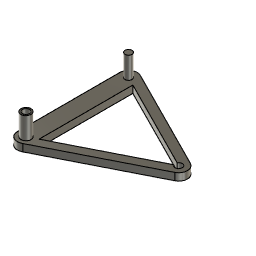
escapement_linkage v6 (Autodesk Fusion 360 archive; units mm, degrees)
design "frame"
Autodesk Fusion 360 part; units mm, degrees
sketch "Sketch1" plane through (0, 0, 0) normal (0, 0, 1) x (1, 0, 0)
  circle A0 centre (0, 0) radius 50
  circle A1 centre (0, 0) radius 37.5
  circle A2 centre (0, 0) radius 33
  circle A3 centre (0, 0) radius 10
  circle A4 centre (0, 0) radius 3.5
  line L0 (0, 0) -> (-100.3747, 100.3747)
  line L1 (0, 0) -> (141.9513, 0) construction
  line L2 (0, 0) -> (0, 143.4713)
  line L3 (-35.3553, 35.3553) -> (13.4462, 84.1569)
  circle A5 centre (0, 70.7107) radius 6
  circle A6 centre (0, 70.7107) radius 2.5
  circle A7 centre (0, 120.7107) radius 6
  line L4 (5.9996, 70.7836) -> (5.9996, 120.7836)
  line L5 (-5.9996, 70.7836) -> (-5.9996, 120.7836)
  line L6 (0, 0) -> (-100.7319, 104.311)
  line L7 (5.9996, 120.7836) -> (5.9996, 95.7836)
  line L8 (-3.0629, 75.87) -> (-47.5954, 50.1551)
  line L9 (-46.505, 50.7838) -> (-53.2901, 46.8719)
  line L10 (46.505, 50.7838) -> (53.2901, 46.8719)
  line L11 (3.0629, 75.87) -> (49.2585, 49.2366)
  line L12 (-53.2901, 46.8719) -> (-50.2933, 41.6739)
  line L13 (-50.2933, 41.6739) -> (0, 64.7107)
  line L14 (50.2933, 41.6739) -> (0, 64.7107)
  line L15 (53.2901, 46.8719) -> (50.2933, 41.6739)
  line L16 (-35.3553, 35.3553) -> (55, 35.3553)
  line L17 (-35.3553, 35.3553) -> (-52, 35.3553)
  line L18 (35.3553, 35.3553) -> (35.3553, 40.6)
  line L19 (35.3553, 35.3553) -> (35.3553, 30.1107)
  line L20 (0, 0) -> (-100.7319, 104.311)
  line L21 (0, 0) -> (-105.6852, 95.1594)
  line L22 (0, 0) -> (142.2568, 0) construction
  circle A8 centre (0, 70.7107) radius 52.618
  circle A9 centre (0, 70.7107) radius 49.5405
  circle A10 centre (34.4479, 35.6863) radius 0.4
  line L23 (25.0068, 27.9448) -> (34.6694, 35.3533)
  line L24 (25.0068, 27.9448) -> (0, 0)
  line L25 (0, 0) -> (19.4334, 32.4512)
  spline S0 degree 5 poles (19.4334, 32.4512) (19.6407, 32.3946) (20.0636, 32.2932) (20.7228, 32.1772) (21.6523, 32.0954) (22.9036, 32.1224) (24.2503, 32.2872) (25.6967, 32.596) (27.2397, 33.0445) (28.8713, 33.6208) (30.5824, 34.3122) (32.0089, 34.9483) (33.1088, 35.469) (33.8553, 35.8351) (34.2318, 36.0229) knots 0 0 0 0 0 0 0.1 0.2 0.3 0.4 0.5 0.6 0.7 0.8 0.9 1 1 1 1 1 1
  circle A11 centre (0, 0) radius 2.5
  point P0 (24.6678, 32.3946)
  dimension "d2" = 75
  dimension "d3" = 66
  dimension "d4" = 20
  dimension "d5" = 7
  dimension "d6" = 135
  dimension "d7" = 12
  dimension "d8" = 5
  dimension "d9" = 12
  dimension "d10" = 50
  dimension "d11" = 1
  dimension "d15" = 6
  dimension "d25" = 138
  dimension "d26" = 1
  dimension "d27" = 0.8
  dimension "d28" = 10.909
  dimension "d62" = 5
  constraint coincident A0.centre A1.centre
  constraint concentric A0 A1
  constraint concentric A1 A2
  constraint concentric A2 A3
  constraint concentric A3 A4
  constraint horizontal L1
  constraint vertical L2
  constraint coincident A0 L3.start
  constraint coincident L0 L3.start
  constraint tangent A0 L3
  constraint coincident L3 A5.centre
  constraint coincident L2 A5.centre
  constraint concentric A5 A6
  constraint coincident A5 L4.start
  constraint symmetric L2 L4.start L5.start
  constraint symmetric L2 L4.end L5.end
  constraint parallel L4 L7
  constraint perpendicular L9 L12
  constraint coincident A5 L13.end
  constraint coincident L2 L13.end
  constraint symmetric L2 L9.end L10.end
  constraint symmetric L2 L12.end L14.start
  constraint symmetric L2 L13.end L14.end
  constraint horizontal L16
  constraint horizontal L17
  constraint coincident A0 L18.start
  constraint coincident L16 L18.start
  constraint perpendicular L16 L18
  constraint symmetric L16 L18.start L19.start
  constraint symmetric L16 L18.end L19.end
  constraint horizontal L22
  constraint concentric A6 A8
  constraint concentric A5 A9
  constraint coincident A1 L23.start
  constraint coincident A9 L23.start
  constraint coincident A10 L23.end
  constraint coincident A10 S0.end
  constraint concentric A3 A11
  measures "d2" diameter of A1
  measures "d3" diameter of A2
  measures "d4" diameter of A3
  measures "d5" diameter of A4
  measures "d6" angle of L0 L1
  measures "d7" diameter of A5
  measures "d8" diameter of A6
  measures "d9" diameter of A7
  measures "d10" distance of L4.start L4.end
  measures "d11" angle of L0 L6
  measures "d15" distance of L9.end L12.end
  measures "d25" angle of L21 L22
  measures "d27" diameter of A10
  measures "d28" angle of L24 L25
  measures "d62" diameter of A11
pattern_circular "C-Pattern1" [no effect]
sketch "Sketch3" plane through (0, 0, 0) normal (0, 0, 1) x (1, 0, 0)
  circle A0 centre (80, 70.7107) radius 6
  circle A1 centre (80, 70.7107) radius 2.45
  circle A2 centre (80, -0.0003) radius 6
  line L0 (80, 70.7107) -> (80, -0.0003)
  line L1 (74, 70.7107) -> (74, -0.0003)
  line L2 (86, 67.6807) -> (86, 3.0309)
  circle A3 centre (80, 0) radius 3.5
  circle A4 centre (80, 0) radius 2.5
  circle A5 centre (54, 100) radius 3
  line L3 (80, 70.7107) -> (80, 35.3607)
  line L4 (150, 35.3607) -> (150, 47)
  line L5 (152.7047, 40.7165) -> (82.7047, 76.0665)
  line L6 (152.7047, 30.0049) -> (82.7047, -5.3451)
  circle A6 centre (150, 35.3607) radius 2.5
  line L7 (150, 47) -> (150, 32.8607)
  line L8 (150, 28.639) -> (150, 24)
  arc A7 (152.7047, 30.0049) -> (152.7047, 40.7165) centre (150, 35.3607) ccw
  line L9 (80, 35.3607) -> (86, 35.3607)
  line L10 (147.5, 35.3607) -> (150, 35.3607)
  line L11 (150, 35.3607) -> (86, 67.6807)
  line L12 (85.3558, 68.006) -> (80, 70.7107)
  line L13 (80, 0) -> (85.3554, 2.7053)
  line L14 (86, 3.0309) -> (150, 35.3607)
  point P0 (0, 70.7107)
  dimension "d68" = 12
  dimension "d71" = 4.9
  dimension "d73" = 12
  dimension "d76" = 6
  dimension "d82" = 7
  dimension "d83" = 5
  dimension "d102" = 6
  dimension "d116" = 12
  dimension "d118" = 5
  constraint vertical L0
  constraint coincident A0.centre A1.centre
  constraint parallel L0 L3
  constraint horizontal L9
  constraint coincident A3.centre A4.centre
  constraint coincident L4.start A6.centre
  constraint perpendicular L4 L9
  constraint perpendicular L7 L9
  constraint symmetric L5.start L6.start L9
  constraint symmetric L5.end L6.end L9
  constraint concentric A6 A7
  constraint coincident L6 L8.start
  constraint collinear L7 L8
  constraint coincident A6 L7.end
  constraint coincident L2 L9.end
  constraint coincident A6 L10.start
  constraint collinear L9 L10
  constraint parallel L0 L2
  constraint coincident A0 L12.start
  constraint collinear L11 L12
  constraint coincident A2 L13.end
  constraint collinear L13 L14
  measures "d68" diameter of A0
  measures "d71" diameter of A1
  measures "d73" diameter of A2
  measures "d82" diameter of A3
  measures "d83" diameter of A4
  measures "d102" diameter of A5
  measures "d116" diameter of A7
  measures "d118" diameter of A6
extrude "Extrude17" add sketch "Sketch3" along normal blind 20 contours A1 L0 L3 L12 | A1 L0 L3 L12 makes body 1
extrude "Extrude18" add sketch "Sketch3" along normal blind 5 contours A0 A1 L0 L3 L12 | A0 A1 L0 L3 L12 bodies 1
extrude "Extrude19" add sketch "Sketch3" along normal blind 5 contours A2 L0 A3 L13 | A2 L0 A3 L13 bodies 1 makes body 2
extrude "Extrude20" add sketch "Sketch3" along normal blind 20 contours L0 A3 A4 L13 | L0 A3 A4 L13 bodies 1 2
extrude "Extrude21" add sketch "Sketch3" along normal blind 10 contours L0 A4 L13 | L0 A4 L13 bodies 2
sketch "Sketch5" plane through (36, 89, 20) normal (0, 0, 1) x (1, 0, 0)
  circle A0 centre (0, 0) radius 3
  dimension "d108" = 6
  constraint coincident A0.centre origin
  measures "d108" diameter of A0
extrude "Extrude15" add sketch "Sketch3" along normal blind 20 separate body contours A1 L0 L3 L12 | A1 L0 L3 L12 makes body 3
extrude "Extrude16" add sketch "Sketch3" along normal blind 5 contours A0 A1 L0 L3 L12 | A0 A1 L0 L3 L12 bodies 3
form "Form1" [no effect]
extrude "Extrude23" add sketch "Sketch3" along normal blind 5 contours A0 L0 L2 L3 L4 L5 A6 L7 L9 L11 | A0 A2 L0 L1 L3 | A2 L0 L2 L4 L5 L6 A6 L7 A7 L9 L14 bodies 1 2 3
